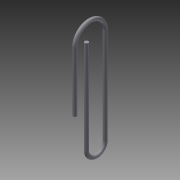
# Autodesk Inventor part: Paperclip
Saved by Autodesk Inventor 2015 (Build 190159000, 159)
## iProperties
Created: 2015-02-13
Part Number: Paperclip
Material: Generic
Document SubType Name: Modeling
Designer: PLTW-Stu-02
Density: 1 g/cm^3
Appearance: Default
Author: PLTW-Stu-02
Autodesk Inventor part; units mm, degrees
ref_plane "YZ Plane" through (0, 0, 0) normal (1, 0, 0) x (0, 1, 0)
ref_plane "XZ Plane" through (0, 0, 0) normal (0, 1, 0) x (-1, 0, 0)
ref_plane "XY Plane" through (0, 0, 0) normal (0, 0, 1) x (1, 0, 0)
sketch "Sketch7" plane through (0, 0, 0) normal (0, 1, 0) x (-1, 0, 0)
  circle A0 centre (0, 0) radius 0.127
  dimension "d2" = 0.254
  constraints: 1 centre point, 1 coincident
  measures "d2" diameter of A0
sketch "Sketch8" plane through (0, 0, 0) normal (1, 0, 0) x (0, 1, 0)
  line L0 (0, 0) -> (4.0856, 0)
  arc A0 (4.0856, -2.1039) -> (4.0856, 0) centre (4.0856, -1.0519) ccw
  line L1 (4.0856, -2.1039) -> (-2.5063, -2.1039)
  arc A1 (-2.4697, -0.8108) -> (-2.5063, -2.1039) centre (-2.5063, -1.4568) ccw
  line L2 (-2.4697, -0.8108) -> (3.9759, -0.8108)
  constraints: 6 end point, 4 point on circle, 3 horizontal, 2 centre point, 2 tangent
sweep "Sweep1" add profiles "Sketch7" path "Sketch8"
body "Solid1"
